Autodesk Fusion 360 part; units mm, degrees
(part 5 of 5)
equation "MountSlotRadius = 0.2 in"
equation "MountSlotLength = 0.551 in"
equation "d12_1 = MountCounterBoreDiameter"
equation "d14_1 = MountSlotLength"
equation "d15_1 = MountSlotRadius"
equation "d24_1 = BoardWidth"
equation "d25_1 = BoardLength"
equation "HoldHoleDiameter = 0.75 in"
equation "d27_1 = HoldHoleDiameter"
equation "d29_1 = MountFirstRowOffset"
equation "d30_1 = HoldDownFirstRowOffset"
equation "HoldFeatureSpacing = 2 in"
equation "BoardWidthCount = 48"
equation "BoardLengthCount = 97"
equation "d44 = BoardWidth / 2 - HoldHoleDiameter"
equation "d45 = CrossMemberSpacing - ( ( MountFirstRowOffset + MountCounterBoreDiameter * 1.25 ) * 1.25 )"
equation "HoldDownFirstRowOffset = MountFirstRowOffset + MountCounterBoreDiameter * 1.25"
equation "HoldDownArrayExtent = 2000 mm"
equation "d49 = NumberOfCrossMembers - 1"
equation "d51 = HoldDownArrayExtent"
equation "d52 = SlotFirstRowOffset"
equation "SlotFirstRowOffset = HoldDownFirstRowOffset * 1.8"
equation "SlotLength = 2.6 in"
equation "d56 = SlotRadius"
equation "SlotRadius = 20 mm"
equation "d58 = SlotLength"
equation "d61 = BoardWidth / 2 - SlotLength"
equation "d64 = SlotLength"
equation "d65 = SlotRadius"
equation "d69 = SlotRadius"
equation "d79 = NumberOfCrossMembers - 1"
equation "d81 = CrossMemberSpacing"
equation "BoardThickness = 0.75 in"
equation "d85 = MountFeaturesPerRow"
equation "d86 = NumberOfCrossMembers"
equation "d87 = BoardWidth / 2 - MountCounterBoreDiameter"
equation "d88 = CrossMemberSpacing * NumberOfCrossMembers"
equation "d100 = NumberOfCrossMembers"
equation "d102 = CrossMemberSpacing"
equation "d103 = BoardThickness"
equation "d105 = BoardThickness - 0.35 in"
equation "d107 = BoardThickness"
equation "d109 = BoardThickness"
equation "d111 = 1\""
equation "d112 = 1/4\""
equation "d113 = 6 3/4\""
equation "d114 = 10\""
equation "d115 = 8\""
equation "d116 = 1/4\""
equation "d118 = 3/4\""
equation "d119 = 38\""
equation "d120 = 3/4\""
equation "d121 = 3/4\""
equation "d122 = 70\""
equation "d123 = 3/4\""
equation "d124 = 90\""
equation "d126 = 1\""
equation "d127 = 10\""
equation "d128 = 1/4\""
equation "d129 = 8\""
equation "d130 = 1/4\""
equation "d131 = 3/4\""
equation "d133 = 3/4\""
equation "d134 = 38\""
equation "d135 = 3/4\""
equation "d137 = 3/4\""
equation "d138 = 90\""
equation "d139 = 1\""
equation "d143 = 1/8\""
equation "d144 = 1/8\""
equation "d145 = 1/8\""
equation "d146 = 1/8\""
equation "d153 = -1/8\""
equation "d157 = 1/8\""
equation "d158 = 1/8\""
equation "d161 = 1/8\""
equation "d163 = 1/8\""
equation "d165 = 1/8\""
